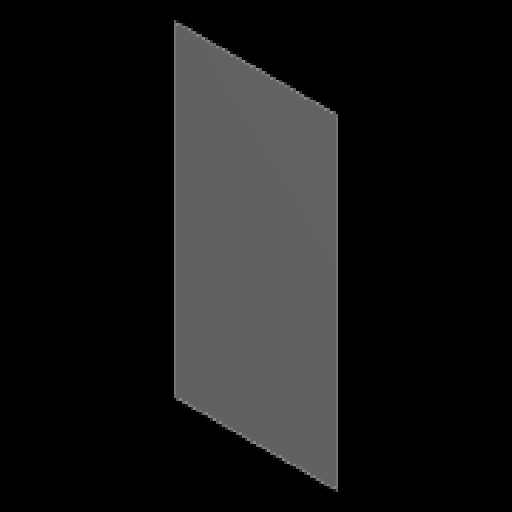
# Autodesk Inventor part: Cart Wheel
Saved by Autodesk Inventor 2025 (Build 290162000, 162)
## iProperties
Created: 2025-03-04
Part Number: Cart Wheel
Material: Generic
Document SubType Name: Modeling
Designer: Trevor
Density: 1 g/cm^3
Appearance: Default
Author: Trevor
Autodesk Inventor part; units mm, degrees
ref_plane "YZ Plane" through (0, 0, 0) normal (1, 0, 0) x (0, 1, 0)
ref_plane "XZ Plane" through (0, 0, 0) normal (0, 1, 0) x (-1, 0, 0)
ref_plane "XY Plane" through (0, 0, 0) normal (0, 0, 1) x (1, 0, 0)
ref_plane "Work Plane1" through (0, 0, 0.2032) normal (0, 0, 1) x (1, 0, 0)
sketch "Sketch1" plane through (0, 0, 0.2032) normal (0, 0, 1) x (1, 0, 0)
  circle A0 centre (-38.1, 25.4) radius 6.35 construction
  circle A1 centre (-38.1, -25.4) radius 6.35 projected
  circle A2 centre (-38.1, 25.4) radius 6.35 construction
  circle A3 centre (-38.1, 25.4) radius 6.55
  circle A4 centre (-38.1, 25.4) radius 19.05 construction
  circle A5 centre (-38.1, 25.4) radius 19.05
  point P0 (0, 0)
  dimension "d0" = 0.2
  constraints: 2 centre point, 1 coincident, 1 concentric
  measures "d0" radial gap between concentric circles of A0 A3
ref_plane "Work Plane2" through (-44.45, 19.05, 25.4) normal (0, 0, 1) x (1, 0, 0)
ref_plane "Work Plane3" through (-48.5775, -83.82, 6.35) normal (0, 0, 1) x (1, 0, 0)
extrude "Extrusion1" add sketch "Sketch1" along normal up to surface (6.1468 mm away) contours A5
sketch "Sketch2" plane through (-38.1, 25.4, 6.35) normal (0, 0, 1) x (1, 0, 0)
  circle A0 centre (0, 0) radius 6.55 projected
  circle A1 centre (0, 0) radius 19.05 projected
  circle A2 centre (0, 0) radius 16.51
  point P0 (38.1, -25.4)
  dimension "d3" = 2.54
  constraints: 1 centre point
  measures "d3" radial gap between concentric circles of A1 A2
ref_plane "Work Plane4" through (-45.085, 18.415, 12.9) normal (0, 0, 1) x (1, 0, 0)
extrude "Extrusion2" add sketch "Sketch2" along normal up to surface (6.55 mm away) contours A2
sketch "Sketch3" plane through (-38.1, 25.4, 12.9) normal (0, 0, 1) x (1, 0, 0)
  circle A0 centre (0, 0) radius 6.55 projected
  circle A1 centre (0, 0) radius 16.51 projected
  circle A2 centre (0, 0) radius 19.05 projected
  circle A3 centre (0, 0) radius 16.51 projected
  circle A4 centre (0, 0) radius 19.05 projected
  point P0 (38.1, -25.4)
ref_plane "Work Plane5" through (-44.45, 19.05, 19.25) normal (0, 0, 1) x (1, 0, 0)
ref_plane "Work Plane6" through (-44.45, 19.05, 19.25) normal (0, 0, 1) x (1, 0, 0)
extrude "Extrusion3" add sketch "Sketch3" along normal up to surface (6.35 mm away) contours A1 | A2
body "Solid1"
